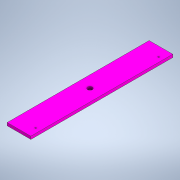
# Autodesk Inventor part: Estabilizador
Saved by Autodesk Inventor 2022 (Build 260153000, 153)
## iProperties
Created: 2022-03-01
Part Number: Estabilizador
Material: Generic
Document SubType Name: Modeling
Designer: Home
Density: 1 g/cm^3
Appearance: Default
Author: Home
Autodesk Inventor part; units mm, degrees
ref_plane "YZ Plane" through (0, 0, 0) normal (1, 0, 0) x (0, 1, 0)
ref_plane "XZ Plane" through (0, 0, 0) normal (0, 1, 0) x (-1, 0, 0)
ref_plane "XY Plane" through (0, 0, 0) normal (0, 0, 1) x (1, 0, 0)
sketch "Sketch1" plane through (0, 0, 0) normal (0, 1, 0) x (-1, 0, 0)
  circle A0 centre (0, 0) radius 5
  line L0 (25, 150) -> (-25, 150)
  line L1 (-25, 150) -> (-25, -150)
  line L2 (-25, -150) -> (25, -150)
  line L3 (25, -150) -> (25, 150)
  line L4 (25, 150) -> (-25, -150) construction
  line L5 (-25, 150) -> (25, -150) construction
  circle A1 centre (-15, 130) radius 1.5
  circle A2 centre (-15, -130) radius 1.5
  dimension "d0" = 10
  dimension "d6" = 50
  dimension "d7" = 300
  dimension "d15" = 3
  dimension "d16" = 10
  dimension "d17" = 3
  dimension "d20" = 20
  dimension "d21" = 20
  constraints: 12 end point, 3 centre point, 2 midpoint, 2 parallel, 1 coincident, 1 horizontal, 1 perpendicular, 1 vertical alignment
  measures "d0" diameter of A0
  measures "d6" distance of L2.end L1.end
  measures "d7" distance of L1.end L0.end
  measures "d15" diameter of A1
  measures "d16" distance from line of A1.centre L1
  measures "d17" diameter of A2
  measures "d20" distance from line of L0 A1.centre
  measures "d21" distance from line of L2 A2.centre
extrude "Extrusion2" add sketch "Sketch1" along normal blind 6
equation "\"d21\" = d20"
body "Solid2"
